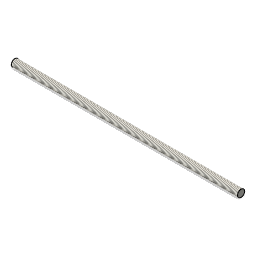
Lead+Screw (Autodesk Fusion 360 design; units mm, degrees)
Autodesk Fusion 360 part; units mm, degrees
note: some values were not read from the file. Set by a fixed rule: which face or edge a step refers to.
sketch "Sketch1" plane through (0, 0, 0) normal (1, 0, 0) x (0, 0, -1)
  circle A0 centre (0, 0) radius 4
  dimension "d1" = 8
  constraint coincident A0.centre origin
  measures "d1" diameter of A0
extrude "Extrude1" add sketch "Sketch1" along normal blind 125 and the other way blind 125
thread "Thread1" "ISO Metric profile 8.0 M8x1.25 6g" major diameter 7.866 minor diameter 6.4455 pitch 1.25 angle 60 resizes the face on face at (83.3333, -0.1994, -3.995) on face at (-83.3333, -0.1994, -3.995)
